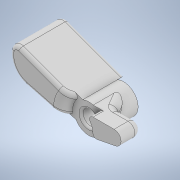
# Autodesk Inventor part: Brazo Sensor
Saved by Autodesk Inventor 2021 (Build 250183000, 183)
## iProperties
Created: 2021-08-27
Part Number: Brazo Sensor
Material: Genérico
Document SubType Name: Modeling
Designer: Diego.labarca
Density: 1 g/cm^3
Appearance: Valor por defecto
Author: Diego.labarca
Autodesk Inventor part; units mm, degrees
ref_plane "YZ Plane" through (0, 0, 0) normal (1, 0, 0) x (0, 1, 0)
ref_plane "XZ Plane" through (0, 0, 0) normal (0, 1, 0) x (-1, 0, 0)
ref_plane "XY Plane" through (0, 0, 0) normal (0, 0, 1) x (1, 0, 0)
sketch "Boceto3" plane through (0, 0, 0) normal (0, 0, 1) x (1, 0, 0)
  circle A0 centre (0, 0) radius 1.1
  circle A1 centre (0, 0) radius 2.1
  line L0 (0, -2.1) -> (5, -2.1) construction
  dimension "d26" = 4.2
  dimension "d25" = 2.2
  constraints: 2 coincident, 2 end point, 1 centre point, 1 horizontal, 1 vertical alignment, 2 other
  measures "d25" diameter of A0
extrude "Extrusión3" add sketch "Boceto3" along normal mid plane 5
ref_plane "Plano de trabajo2" through (0, 0, 4) normal (0, 0, 1) x (1, 0, 0)
sketch "Boceto8" plane through (0, 0, 4) normal (0, 0, 1) x (1, 0, 0)
  circle A0 centre (0, 0) radius 2.1 projected
  line L0 (2.0396, -0.5) -> (6.5396, -0.5)
  line L1 (6.5396, -0.5) -> (6.5396, 2)
  line L2 (6.5396, 2) -> (0.6403, 2)
  dimension "d58" = 4.5
  dimension "d59" = 2.5
  dimension "d60" = 0.5
  constraints: 6 end point, 2 perpendicular, 2 point on circle, 1 horizontal
  measures "d58" distance of L0.start L0.end
  measures "d59" distance of L0.end L1.end
  measures "d60" vertical distance of L0.start point (0, 0)
extrude "Extrusión8" add sketch "Boceto8" against normal blind 3 contours A0 L2 L1 L0
sketch "Boceto9" plane through (0.6403, 2, 4) normal (0, 1, 0) x (1, 0, 0)
  line L0 (1.4597, 3) -> (0, 3) projected
  line L1 (0, 3) -> (0, 6.5)
  line L2 (1.4597, 6.5) -> (-2.7403, 6.5) projected
  line L3 (0, 6.5) -> (2.0207, 3)
  line L4 (0, 3) -> (5.8993, 3) projected
  line L5 (0, 6.5) -> (4.0415, 6.5) construction
  line L6 (2.0207, 3) -> (0, 3)
  point P0 (-0.6403, 4)
  point P1 (1.3993, 3)
  dimension "d71" = 60
  constraints: 8 end point, 2 point on line, 1 collinear, 1 equal length, 1 horizontal, 1 vertical
  measures "d71" angle of L3 L5
extrude "Extrusión9" add sketch "Boceto9" against normal up to surface (2.5 mm away)
sketch "Boceto11" plane through (0, 0, -2.5) normal (0, 0, -1) x (-1, 0, 0)
  line L0 (-2.661, 2) -> (-6.5396, 2) projected
  line L1 (-6.5396, 2) -> (-6.5396, -0.5) projected
  line L2 (-6.5396, -0.5) -> (-2.661, -0.5) projected
  line L3 (-6.5396, 2) -> (-6.5396, -0.5) projected
  line L4 (-6.5396, -0.5) -> (-3.5707, -0.5) projected
  line L5 (-6.5396, -0.5) -> (-6.5396, 0.25)
  line L6 (-2.661, -0.5) -> (-2.661, 2) projected
  line L7 (-2.661, -0.5) -> (-2.0396, -0.5) projected
  line L8 (-6.5396, 0.25) -> (-2.661, -0.5)
  line L9 (-2.661, -0.5) -> (-6.5396, -0.5)
  point P0 (0, 0)
  dimension "d104" = 0.75
  constraints: 6 end point, 1 collinear, 1 point on line
  measures "d104" distance of L1.end L5.end
extrude "Extrusión11" cut sketch "Boceto11" against normal up to surface (6.5 mm away) contours L2 L1 L8
sketch "Boceto12" plane through (0, 0, -2.5) normal (0, 0, -1) x (-1, 0, 0)
  circle A0 centre (0, 0) radius 1.1 projected
  point P0 (-0.6403, 0.8944)
  constraints: 1 other
extrude "Extrusión12" cut sketch "Boceto12" against normal up to surface (5 mm away)
ref_plane "Plano de trabajo5" through (0, 0, 3.5) normal (0, 0, 1) x (1, 0, 0)
sketch "Boceto13" plane through (0, 0, 3.5) normal (0, 0, 1) x (1, 0, 0)
  circle A0 centre (0, 0) radius 2.1 projected
  line L0 (-1.8508, 0.9922) -> (3.1492, 0.9922) construction
  line L1 (-2, 0) -> (8, 0) construction
  line L2 (-11.2314, 1.4313) -> (-9.8633, 5.1901)
  line L3 (-9.8633, 5.1901) -> (-0.8633, 1.9143)
  line L4 (-11.2314, 1.4313) -> (-7.91, 1.4313) construction
  arc A1 (2.0396, -0.5) -> (0.6403, 2) centre (0, 0) ccw projected
  arc A2 (0.6403, 2) -> (2.0396, -0.5) centre (0, 0) ccw projected
  circle A3 centre (0, 0) radius 2.1 projected
  line L5 (-11.2314, 1.4313) -> (-1.8325, -1.0257)
  arc A4 (0.6403, 2) -> (2.0396, -0.5) centre (0, 0) ccw projected
  line L6 (0, 2.1) -> (0, 2.7078)
  point P0 (-0.8633, 1.9143)
  point P1 (-1.8325, -1.0257)
  dimension "d98" = 4
  dimension "d120" = 9
  dimension "d139" = 70
  constraints: 14 end point, 3 horizontal, 2 point on circle, 1 perpendicular, 1 vertical, 7 other
  measures "d98" distance of L2.start L2.end
  measures "d120" horizontal distance of L2.end L3.end
  measures "d139" angle of L6 L3
extrude "Extrusión13" add sketch "Boceto13" against normal blind 7 contours L5 L2 L3 A0
fillet "Empalme20" radius 3 1 edges at (-11.2314, 1.4313, 0)
sketch "Boceto18" plane through (0, 0, -3.5) normal (0, 0, -1) x (-1, 0, 0)
  line L0 (0.8633, 1.9143) -> (9.8633, 5.1901) projected
  line L1 (9.1116, 4.9165) -> (9.3852, 4.1647)
  line L2 (9.1116, 4.9165) -> (9.9116, 4.9165) construction
  line L3 (9.3852, 4.1647) -> (3.5591, 2.0442)
  line L4 (3.5591, 2.0442) -> (3.9695, 0.9165)
  line L5 (3.9695, 0.9165) -> (9.7956, 3.0371)
  line L6 (9.7956, 3.0371) -> (9.3852, 4.1647)
  point P0 (0, 0)
  dimension "d122" = 0.8
  dimension "d123" = 70
  dimension "d124" = 6.2
  dimension "d125" = 1.2
  dimension "d141" = 90
  constraints: 12 end point, 4 perpendicular, 1 equal length, 1 horizontal, 1 point on line
  measures "d122" distance of L1.start L1.end
  measures "d123" angle of L1 L2
  measures "d124" distance of L1.end L3.end
  measures "d125" distance of L3.end L4.end
  measures "d141" angle of L3 L6
extrude "Extrusión16" cut sketch "Boceto18" against normal blind 6.6
fillet "Empalme21" radius 1 1 edges at (-9.8633, 5.1901, 0)
fillet "Empalme23" radius 0.5 2 edges at (0.6403, 2, 3.25) (2.0396, -0.5, 3.25)
fillet "Empalme24" radius 0.5 1 edges at (2.661, 0.75, 1)
fillet "Empalme28" radius 1 2 edges at (6.5396, 2, 2.5) (6.5396, 0.25, 2.5)
sketch "Boceto20" plane through (0, 0, 3.5) normal (0, 0, 1) x (1, 0, 0)
  circle A0 centre (0, 0) radius 2.3
  dimension "d145" = 4.6
  constraints: 1 centre point, 1 coincident
  measures "d145" diameter of A0
extrude "Extrusión18" cut sketch "Boceto20" against normal up to surface (1 mm away)
fillet "Empalme29" radius 2 1 edges at (-2.1861, 0.7147, 3.5)
fillet "Empalme31" radius 3 2 edges at (-3.7643, 1.4804, 3.1) (-9.5904, 3.6009, 3.1)
fillet "Empalme32" radius 1 6 edges at (2.7983, -0.4735, 0.9765) (6.1464, 1.0954, 1) (4.0503, 2, 1) (2.6997, 2, 0.933) (1.5785, 2, -0.875) (4.1453, -0.213, 1)
fillet "Empalme33" radius 0.5 8 edges at (-4.9384, -0.2137, -3.5) (-4.8833, 3.3775, -3.5) (-9.7335, 4.7736, 3.5) (-5.9523, 3.7666, 3.5) (-1.9525, 2.3108, 3.2281) (-6.0252, 0.0703, 3.5) (-2.935, -0.7375, 3.2287) (-9.8325, 1.9152, 3.5)
fillet "Empalme34" radius 0.3 5 edges at (-0.5028, 0.9784, -2.5) (0, -1.1, -2.5) (0.9784, 0.5028, -2.5) (0, 1.1, 2.5) (0, -1.1, 2.5)
